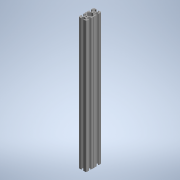
# Autodesk Inventor part: Gantry Cross Beam
Saved by Autodesk Inventor 2022.3 (Build 263350000, 350)
## iProperties
Category: PARTsolutions
Company: 8020
Part Number: Gantry Cross Beam
Material: Generic
Catalog Web Link: www.cadenas.de
Description: 1530, 1530-Black, 1530-Black-FB-T-Slotted Profile - 15 Series
Vendor: 8020
Document SubType Name: Modeling
Designer: partserver
Manufacturer: 8020
Mass: 68.215 g
Surface Area: 329.489 cm^2
Volume: 68.215 cm^3
Density: 1 g/cm^3
Appearance: PSOLRGB-191-191-191
PSOL_IDENT_0: {$CADENAS_DATA\23d-libs\8020\inch\profiles\15_series\1530.prj},192 {VTYP=3D},{NB=1530-2-CL},{LINA=15
PSOL_IDENT_1: 30-2},{NN=1530, 1530-Black, 1530-Black-FB},{DATE=31.07.2020 09:21:23},{GEOMDATE=09.02.2018 15:56:31}
PSOL_IDENT_2: ,{VERSION=},{LINEID=10},{WBVAR=FINISH,LS,L},{WBNUMERIC=L}  {NB=1530-2-CL},{LINA=1530-2},{KT=DUMMY},{
PSOL_IDENT_3: PN=1530-2},{SERIES=1530},{MAT=6105-T5 Aluminum},{FINISH=CA},{LS=-CL},{L=2.000},{LALG=[1:242/0.005]},
PSOL_IDENT_4: {W=2.4209},{MIX=1.8042},{MIY=.4824},{EA=2.0798},{CLR=.75,.75,.75}
NB: 1530-2-CL
NN: 1530, 1530-Black, 1530-Black-FB
NT: T-Slotted Profile - 15 Series
NBSYN: $PN.$LS.
LINA: 1530-2
CATALOG: 80/20
PN: 1530-2
SERIES: 1530
MAT: 6105-T5 Aluminum
FINISH: Clear Anodize
LS: Custom Length
L: 2
W: 2.4209
MIX: 1.8042
MIY: .4824
EA: 2.0798
SUPPLIER: 8020
ARTICLENO: 1530-2-CL
BOMINFO: 1530-2
CREATOR: CADENAS GmbH
Title: 1530-2
Author: Cadenas PARTsolutions
Comments: T-Slotted Profile - 15 Series
Autodesk Inventor part; units mm, degrees
sketch "Sketch_1" plane through (0, 0, 0) normal (0, 0, 1) x (1, 0, 0)
  arc A0 (-15.8496, 57.15) -> (-19.05, 53.9496) centre (-15.8751, 53.9751) ccw
  arc A1 (-19.05, 52.4256) -> (-19.05, 53.9496) centre (-19.05, 53.1876) ccw
  line L0 (-19.05, 52.4256) -> (-19.05, 47.5996)
  arc A2 (-19.05, 46.0756) -> (-19.05, 47.5996) centre (-19.05, 46.8376) ccw
  line L1 (-19.05, 46.0756) -> (-19.05, 43.7388)
  arc A3 (-19.05, 43.7388) -> (-17.4752, 42.164) centre (-17.4752, 43.7388) ccw
  line L2 (-17.4752, 42.164) -> (-16.5608, 42.164)
  arc A4 (-16.5608, 42.164) -> (-14.986, 43.7388) centre (-16.5608, 43.7388) ccw
  line L3 (-14.986, 43.7388) -> (-14.986, 47.498)
  arc A5 (-14.097, 48.387) -> (-14.986, 47.498) centre (-14.097, 47.498) ccw
  line L4 (-14.097, 48.387) -> (-13.5289, 48.387)
  arc A6 (-12.9003, 48.1266) -> (-13.5289, 48.387) centre (-13.5289, 47.498) ccw
  line L5 (-12.9003, 48.1266) -> (-8.1476, 43.3739)
  arc A7 (-6.7564, 40.0153) -> (-8.1476, 43.3739) centre (-11.5062, 40.0153) ccw
  line L6 (-6.7564, 40.0153) -> (-6.7564, 36.1847)
  arc A8 (-8.1476, 32.8261) -> (-6.7564, 36.1847) centre (-11.5062, 36.1847) ccw
  line L7 (-8.1476, 32.8261) -> (-12.9003, 28.0734)
  arc A9 (-13.5289, 27.813) -> (-12.9003, 28.0734) centre (-13.5289, 28.702) ccw
  line L8 (-13.5289, 27.813) -> (-14.097, 27.813)
  arc A10 (-14.986, 28.702) -> (-14.097, 27.813) centre (-14.097, 28.702) ccw
  line L9 (-14.986, 28.702) -> (-14.986, 32.4612)
  arc A11 (-14.986, 32.4612) -> (-16.5608, 34.036) centre (-16.5608, 32.4612) ccw
  line L10 (-16.5608, 34.036) -> (-17.4752, 34.036)
  arc A12 (-17.4752, 34.036) -> (-19.05, 32.4612) centre (-17.4752, 32.4612) ccw
  line L11 (-19.05, 32.4612) -> (-19.05, 30.1244)
  arc A13 (-19.05, 28.6004) -> (-19.05, 30.1244) centre (-19.05, 29.3624) ccw
  line L12 (-19.05, 28.6004) -> (-19.05, 23.7744)
  arc A14 (-19.05, 22.2504) -> (-19.05, 23.7744) centre (-19.05, 23.0124) ccw
  line L13 (-19.05, 22.2504) -> (-19.05, 15.8496)
  arc A15 (-19.05, 14.3256) -> (-19.05, 15.8496) centre (-19.05, 15.0876) ccw
  line L14 (-19.05, 14.3256) -> (-19.05, 9.4996)
  arc A16 (-19.05, 7.9756) -> (-19.05, 9.4996) centre (-19.05, 8.7376) ccw
  line L15 (-19.05, 7.9756) -> (-19.05, 5.6388)
  arc A17 (-19.05, 5.6388) -> (-17.4752, 4.064) centre (-17.4752, 5.6388) ccw
  line L16 (-17.4752, 4.064) -> (-16.5608, 4.064)
  arc A18 (-16.5608, 4.064) -> (-14.986, 5.6388) centre (-16.5608, 5.6388) ccw
  line L17 (-14.986, 5.6388) -> (-14.986, 9.398)
  arc A19 (-14.097, 10.287) -> (-14.986, 9.398) centre (-14.097, 9.398) ccw
  line L18 (-14.097, 10.287) -> (-13.5289, 10.287)
  arc A20 (-12.9003, 10.0266) -> (-13.5289, 10.287) centre (-13.5289, 9.398) ccw
  line L19 (-12.9003, 10.0266) -> (-8.1476, 5.2739)
  arc A21 (-6.7564, 1.9153) -> (-8.1476, 5.2739) centre (-11.5062, 1.9153) ccw
  line L20 (-6.7564, 1.9153) -> (-6.7564, -1.9153)
  arc A22 (-8.1476, -5.2739) -> (-6.7564, -1.9153) centre (-11.5062, -1.9153) ccw
  line L21 (-8.1476, -5.2739) -> (-12.9003, -10.0266)
  arc A23 (-13.5289, -10.287) -> (-12.9003, -10.0266) centre (-13.5289, -9.398) ccw
  line L22 (-13.5289, -10.287) -> (-14.097, -10.287)
  arc A24 (-14.986, -9.398) -> (-14.097, -10.287) centre (-14.097, -9.398) ccw
  line L23 (-14.986, -9.398) -> (-14.986, -5.6388)
  arc A25 (-14.986, -5.6388) -> (-16.5608, -4.064) centre (-16.5608, -5.6388) ccw
  line L24 (-16.5608, -4.064) -> (-17.4752, -4.064)
  arc A26 (-17.4752, -4.064) -> (-19.05, -5.6388) centre (-17.4752, -5.6388) ccw
  line L25 (-19.05, -5.6388) -> (-19.05, -7.9756)
  arc A27 (-19.05, -9.4996) -> (-19.05, -7.9756) centre (-19.05, -8.7376) ccw
  line L26 (-19.05, -9.4996) -> (-19.05, -14.3256)
  arc A28 (-19.05, -15.8496) -> (-19.05, -14.3256) centre (-19.05, -15.0876) ccw
  arc A29 (-19.05, -15.8496) -> (-15.8496, -19.05) centre (-15.8751, -15.8751) ccw
  arc A30 (-14.3256, -19.05) -> (-15.8496, -19.05) centre (-15.0876, -19.05) ccw
  line L27 (-14.3256, -19.05) -> (-9.4996, -19.05)
  arc A31 (-7.9756, -19.05) -> (-9.4996, -19.05) centre (-8.7376, -19.05) ccw
  line L28 (-7.9756, -19.05) -> (-5.6388, -19.05)
  arc A32 (-5.6388, -19.05) -> (-4.064, -17.4752) centre (-5.6388, -17.4752) ccw
  line L29 (-4.064, -17.4752) -> (-4.064, -16.5608)
  arc A33 (-4.064, -16.5608) -> (-5.6388, -14.986) centre (-5.6388, -16.5608) ccw
  line L30 (-5.6388, -14.986) -> (-9.398, -14.986)
  arc A34 (-10.287, -14.097) -> (-9.398, -14.986) centre (-9.398, -14.097) ccw
  line L31 (-10.287, -14.097) -> (-10.287, -13.5289)
  arc A35 (-10.0266, -12.9003) -> (-10.287, -13.5289) centre (-9.398, -13.5289) ccw
  line L32 (-10.0266, -12.9003) -> (-5.2739, -8.1476)
  arc A36 (-1.9153, -6.7564) -> (-5.2739, -8.1476) centre (-1.9153, -11.5062) ccw
  line L33 (-1.9153, -6.7564) -> (1.9153, -6.7564)
  arc A37 (5.2739, -8.1476) -> (1.9153, -6.7564) centre (1.9153, -11.5062) ccw
  line L34 (5.2739, -8.1476) -> (10.0266, -12.9003)
  arc A38 (10.287, -13.5289) -> (10.0266, -12.9003) centre (9.398, -13.5289) ccw
  line L35 (10.287, -13.5289) -> (10.287, -14.097)
  arc A39 (9.398, -14.986) -> (10.287, -14.097) centre (9.398, -14.097) ccw
  line L36 (9.398, -14.986) -> (5.6388, -14.986)
  arc A40 (5.6388, -14.986) -> (4.064, -16.5608) centre (5.6388, -16.5608) ccw
  line L37 (4.064, -16.5608) -> (4.064, -17.4752)
  arc A41 (4.064, -17.4752) -> (5.6388, -19.05) centre (5.6388, -17.4752) ccw
  line L38 (5.6388, -19.05) -> (7.9756, -19.05)
  arc A42 (9.4996, -19.05) -> (7.9756, -19.05) centre (8.7376, -19.05) ccw
  line L39 (9.4996, -19.05) -> (14.3256, -19.05)
  arc A43 (15.8496, -19.05) -> (14.3256, -19.05) centre (15.0876, -19.05) ccw
  arc A44 (15.8496, -19.05) -> (19.05, -15.8496) centre (15.8751, -15.8751) ccw
  arc A45 (19.05, -14.3256) -> (19.05, -15.8496) centre (19.05, -15.0876) ccw
  line L40 (19.05, -14.3256) -> (19.05, -9.4996)
  arc A46 (19.05, -7.9756) -> (19.05, -9.4996) centre (19.05, -8.7376) ccw
  line L41 (19.05, -7.9756) -> (19.05, -5.6388)
  arc A47 (19.05, -5.6388) -> (17.4752, -4.064) centre (17.4752, -5.6388) ccw
  line L42 (17.4752, -4.064) -> (16.5608, -4.064)
  arc A48 (16.5608, -4.064) -> (14.986, -5.6388) centre (16.5608, -5.6388) ccw
  line L43 (14.986, -5.6388) -> (14.986, -9.398)
  arc A49 (14.097, -10.287) -> (14.986, -9.398) centre (14.097, -9.398) ccw
  line L44 (14.097, -10.287) -> (13.5289, -10.287)
  arc A50 (12.9003, -10.0266) -> (13.5289, -10.287) centre (13.5289, -9.398) ccw
  line L45 (12.9003, -10.0266) -> (8.1476, -5.2739)
  arc A51 (6.7564, -1.9153) -> (8.1476, -5.2739) centre (11.5062, -1.9153) ccw
  line L46 (6.7564, -1.9153) -> (6.7564, 1.9153)
  arc A52 (8.1476, 5.2739) -> (6.7564, 1.9153) centre (11.5062, 1.9153) ccw
  line L47 (8.1476, 5.2739) -> (12.9003, 10.0266)
  arc A53 (13.5289, 10.287) -> (12.9003, 10.0266) centre (13.5289, 9.398) ccw
  line L48 (13.5289, 10.287) -> (14.097, 10.287)
  arc A54 (14.986, 9.398) -> (14.097, 10.287) centre (14.097, 9.398) ccw
  line L49 (14.986, 9.398) -> (14.986, 5.6388)
  arc A55 (14.986, 5.6388) -> (16.5608, 4.064) centre (16.5608, 5.6388) ccw
  line L50 (16.5608, 4.064) -> (17.4752, 4.064)
  arc A56 (17.4752, 4.064) -> (19.05, 5.6388) centre (17.4752, 5.6388) ccw
  line L51 (19.05, 5.6388) -> (19.05, 7.9756)
  arc A57 (19.05, 9.4996) -> (19.05, 7.9756) centre (19.05, 8.7376) ccw
  line L52 (19.05, 9.4996) -> (19.05, 14.3256)
  arc A58 (19.05, 15.8496) -> (19.05, 14.3256) centre (19.05, 15.0876) ccw
  line L53 (19.05, 15.8496) -> (19.05, 22.2504)
  arc A59 (19.05, 23.7744) -> (19.05, 22.2504) centre (19.05, 23.0124) ccw
  line L54 (19.05, 23.7744) -> (19.05, 28.6004)
  arc A60 (19.05, 30.1244) -> (19.05, 28.6004) centre (19.05, 29.3624) ccw
  line L55 (19.05, 30.1244) -> (19.05, 32.4612)
  arc A61 (19.05, 32.4612) -> (17.4752, 34.036) centre (17.4752, 32.4612) ccw
  line L56 (17.4752, 34.036) -> (16.5608, 34.036)
  arc A62 (16.5608, 34.036) -> (14.986, 32.4612) centre (16.5608, 32.4612) ccw
  line L57 (14.986, 32.4612) -> (14.986, 28.702)
  arc A63 (14.097, 27.813) -> (14.986, 28.702) centre (14.097, 28.702) ccw
  line L58 (14.097, 27.813) -> (13.5289, 27.813)
  arc A64 (12.9003, 28.0734) -> (13.5289, 27.813) centre (13.5289, 28.702) ccw
  line L59 (12.9003, 28.0734) -> (8.1476, 32.8261)
  arc A65 (6.7564, 36.1847) -> (8.1476, 32.8261) centre (11.5062, 36.1847) ccw
  line L60 (6.7564, 36.1847) -> (6.7564, 40.0153)
  arc A66 (8.1476, 43.3739) -> (6.7564, 40.0153) centre (11.5062, 40.0153) ccw
  line L61 (8.1476, 43.3739) -> (12.9003, 48.1266)
  arc A67 (13.5289, 48.387) -> (12.9003, 48.1266) centre (13.5289, 47.498) ccw
  line L62 (13.5289, 48.387) -> (14.097, 48.387)
  arc A68 (14.986, 47.498) -> (14.097, 48.387) centre (14.097, 47.498) ccw
  line L63 (14.986, 47.498) -> (14.986, 43.7388)
  arc A69 (14.986, 43.7388) -> (16.5608, 42.164) centre (16.5608, 43.7388) ccw
  line L64 (16.5608, 42.164) -> (17.4752, 42.164)
  arc A70 (17.4752, 42.164) -> (19.05, 43.7388) centre (17.4752, 43.7388) ccw
  line L65 (19.05, 43.7388) -> (19.05, 46.0756)
  arc A71 (19.05, 47.5996) -> (19.05, 46.0756) centre (19.05, 46.8376) ccw
  line L66 (19.05, 47.5996) -> (19.05, 52.4256)
  arc A72 (19.05, 53.9496) -> (19.05, 52.4256) centre (19.05, 53.1876) ccw
  arc A73 (19.05, 53.9496) -> (15.8496, 57.15) centre (15.8751, 53.9751) ccw
  arc A74 (14.3256, 57.15) -> (15.8496, 57.15) centre (15.0876, 57.15) ccw
  line L67 (14.3256, 57.15) -> (9.4996, 57.15)
  arc A75 (7.9756, 57.15) -> (9.4996, 57.15) centre (8.7376, 57.15) ccw
  line L68 (7.9756, 57.15) -> (5.6388, 57.15)
  arc A76 (5.6388, 57.15) -> (4.064, 55.5752) centre (5.6388, 55.5752) ccw
  line L69 (4.064, 55.5752) -> (4.064, 54.6608)
  arc A77 (4.064, 54.6608) -> (5.6388, 53.086) centre (5.6388, 54.6608) ccw
  line L70 (5.6388, 53.086) -> (9.398, 53.086)
  arc A78 (10.287, 52.197) -> (9.398, 53.086) centre (9.398, 52.197) ccw
  line L71 (10.287, 52.197) -> (10.287, 51.6289)
  arc A79 (10.0266, 51.0003) -> (10.287, 51.6289) centre (9.398, 51.6289) ccw
  line L72 (10.0266, 51.0003) -> (5.2739, 46.2476)
  arc A80 (1.9153, 44.8564) -> (5.2739, 46.2476) centre (1.9153, 49.6062) ccw
  line L73 (1.9153, 44.8564) -> (-1.9153, 44.8564)
  arc A81 (-5.2739, 46.2476) -> (-1.9153, 44.8564) centre (-1.9153, 49.6062) ccw
  line L74 (-5.2739, 46.2476) -> (-10.0266, 51.0003)
  arc A82 (-10.287, 51.6289) -> (-10.0266, 51.0003) centre (-9.398, 51.6289) ccw
  line L75 (-10.287, 51.6289) -> (-10.287, 52.197)
  arc A83 (-9.398, 53.086) -> (-10.287, 52.197) centre (-9.398, 52.197) ccw
  line L76 (-9.398, 53.086) -> (-5.6388, 53.086)
  arc A84 (-5.6388, 53.086) -> (-4.064, 54.6608) centre (-5.6388, 54.6608) ccw
  line L77 (-4.064, 54.6608) -> (-4.064, 55.5752)
  arc A85 (-4.064, 55.5752) -> (-5.6388, 57.15) centre (-5.6388, 55.5752) ccw
  line L78 (-5.6388, 57.15) -> (-7.9756, 57.15)
  arc A86 (-9.4996, 57.15) -> (-7.9756, 57.15) centre (-8.7376, 57.15) ccw
  line L79 (-9.4996, 57.15) -> (-14.3256, 57.15)
  arc A87 (-15.8496, 57.15) -> (-14.3256, 57.15) centre (-15.0876, 57.15) ccw
  circle A88 centre (0, 0) radius 3.3274
  circle A89 centre (0, 38.1) radius 3.3274
  arc A90 (-14.1109, 21.1155) -> (-14.1109, 16.9845) centre (-12.0454, 19.05) ccw
  line L80 (-14.1109, 16.9845) -> (-5.2739, 8.1476)
  arc A91 (-5.2739, 8.1476) -> (-1.9153, 6.7564) centre (-1.9153, 11.5062) ccw
  line L81 (-1.9153, 6.7564) -> (1.9153, 6.7564)
  arc A92 (1.9153, 6.7564) -> (5.2739, 8.1476) centre (1.9153, 11.5062) ccw
  line L82 (5.2739, 8.1476) -> (14.1109, 16.9845)
  arc A93 (14.1109, 16.9845) -> (14.1109, 21.1155) centre (12.0454, 19.05) ccw
  line L83 (14.1109, 21.1155) -> (5.2739, 29.9524)
  arc A94 (5.2739, 29.9524) -> (1.9153, 31.3436) centre (1.9153, 26.5938) ccw
  line L84 (1.9153, 31.3436) -> (-1.9153, 31.3436)
  arc A95 (-1.9153, 31.3436) -> (-5.2739, 29.9524) centre (-1.9153, 26.5938) ccw
  line L85 (-5.2739, 29.9524) -> (-14.1109, 21.1155)
  constraints: 188 point on circle, 172 end point, 96 centre point
extrude "Extrusion1" add sketch "Sketch_1" against normal blind 647.7
ref_plane "b1_XY" through (0, -19.05, -25.4) normal (0, 1, 0) x (1, 0, 0)
ref_plane "b1_YZ" through (0, -19.05, -25.4) normal (1, 0, 0) x (0, 0, -1)
ref_plane "b1_ZX" through (0, -19.05, -25.4) normal (0, 0, -1) x (0, 1, 0)
ref_plane "b2_XY" through (0, 57.15, -25.4) normal (0, 1, 0) x (1, 0, 0)
ref_plane "b2_YZ" through (0, 57.15, -25.4) normal (1, 0, 0) x (0, 0, -1)
ref_plane "b2_ZX" through (0, 57.15, -25.4) normal (0, 0, -1) x (0, 1, 0)
ref_plane "profile1530_XY" through (0, 19.05, -25.4) normal (0, 0, 1) x (1, 0, 0)
ref_plane "profile1530_YZ" through (0, 19.05, -25.4) normal (1, 0, 0) x (0, 1, 0)
ref_plane "profile1530_ZX" through (0, 19.05, -25.4) normal (0, 1, 0) x (0, 0, 1)
body "Solid1"
